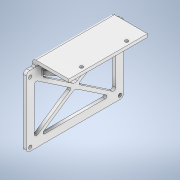
# Autodesk Inventor part: batteryBracket
Saved by Autodesk Inventor 2022 (Build 260153000, 153)
## iProperties
Created: 2022-04-12
Part Number: batteryBracket
Material: PC/ABS Plastic
Document SubType Name: Modeling
Designer: Dahway
Mass: 22.0736 g
Surface Area: 159.209 cm^2
Volume: 22.0736 cm^3
Density: 0.357273 g/cm^3
Appearance: Smooth - White
Author: Dahway
Autodesk Inventor part; units mm, degrees
ref_plane "YZ Plane" through (0, 0, 0) normal (1, 0, 0) x (0, 1, 0)
ref_plane "XZ Plane" through (0, 0, 0) normal (0, 1, 0) x (-1, 0, 0)
ref_plane "XY Plane" through (0, 0, 0) normal (0, 0, 1) x (1, 0, 0)
sketch "Sketch1" plane through (0, 0, 0) normal (0, 1, 0) x (-1, 0, 0)
  line L0 (0, 0) -> (34.8, 0)
  line L1 (34.8, 0) -> (34.8, 75.4)
  line L2 (34.8, 75.4) -> (0, 75.4)
  line L3 (0, 75.4) -> (0, 0)
  dimension "d0" = 34.8
  dimension "d1" = 75.4
  constraints: 8 end point, 2 parallel, 1 horizontal, 1 perpendicular
  measures "d0" distance of L2.end L1.end
  measures "d1" distance of L1.end L0.end
extrude "Extrusion1" add sketch "Sketch1" along normal blind 40.7
sketch "Sketch2" plane through (0, 0, 0) normal (0, -1, 0) x (1, 0, 0)
  line L0 (0, 75.4) -> (0, 0) projected
  line L1 (-34.8, 75.4) -> (0, 75.4) projected
  line L2 (0, 0) -> (-31.8, 0)
  line L3 (-31.8, 0) -> (-31.8, 75.4)
  line L4 (-31.8, 75.4) -> (0, 75.4)
  line L5 (0, 75.4) -> (0, 0)
  dimension "d4" = 31.8
  constraints: 8 end point, 2 parallel, 1 horizontal, 1 perpendicular, 1 point on line
  measures "d4" distance of L3.end L4.end
extrude "Extrusion2" cut sketch "Sketch2" against normal blind 37.7
ref_plane "Work Plane1" through (0, 40.7, 37.7) normal (0, 0, -1) x (-1, 0, 0)
sketch "Sketch4" plane through (0, 37.7, 0) normal (0, -1, 0) x (1, 0, 0)
  circle A0 centre (-4, 3.7) radius 1.5
  circle A1 centre (-4, 6.5) radius 1.5
  line L0 (-5.5, 3.7) -> (-5.5, 6.5)
  line L1 (-2.5, 3.7) -> (-2.5, 6.5)
  line L2 (0, 0) -> (-31.8, 0) projected
  line L3 (0, 75.4) -> (0, 0) projected
  dimension "d17" = 3
  dimension "d18" = 3
  dimension "d19" = 3.7
  dimension "d20" = 4
  dimension "d21" = 2.8
  constraints: 4 end point, 4 point on circle, 2 centre point, 2 tangent, 1 parallel, 1 vertical
  measures "d17" diameter of A0
  measures "d18" diameter of A1
  measures "d19" distance from line of L2 A0.centre
  measures "d20" distance from line of L3 A0.centre
  measures "d21" distance of A1.centre A0.centre
extrude "Extrusion4" add sketch "Sketch4" along normal blind 3
fillet "Fillet1" radius 1 4 edges at (-4, 34.7, 2.2) (-2.5, 34.7, 5.1) (-4, 34.7, 8) (-5.5, 34.7, 5.1)
mirror "Mirror2" about plane through (0, 40.7, 37.7) normal (0, 0, -1) of "Extrusion4", "Fillet1"
sketch "Sketch22" plane through (0, 40.7, 0) normal (0, 1, 0) x (1, 0, 0)
  line L0 (-34.8, -75.4) -> (0, -75.4) projected
  line L1 (-7.8, -72.1) -> (-7.8, -75.4) projected
  line L2 (0, 0) -> (-34.8, 0) projected
  point P0 (-4, -59.3)
  point P1 (-3.9, -16.1)
  point P2 (-7.8, 0)
  dimension "d126" = 16.1
  dimension "d127" = 3.8
  dimension "d128" = 16.1
  measures "d126" distance from line of L0 point (-4, -59.3)
  measures "d127" distance from line of L1 point (-4, -59.3)
  measures "d128" distance from line of L2 point (-3.9, -16.1)
hole "Hole2" at (-4, 40.7, 59.3) at (-3.9, 40.7, 16.1) direction (0, -1, 0) diameter 3.15 depth 3 tip angle 118
sketch "Sketch24" plane through (-34.8, 0, 0) normal (-1, 0, 0) x (0, 0, 1)
  line L0 (84.25, 34.785) -> (-8.85, 34.785)
  line L1 (-8.85, 34.785) -> (-8.85, -32.5)
  line L2 (-8.85, -32.5) -> (84.25, -32.5)
  line L3 (84.25, -32.5) -> (84.25, 34.785)
  point P0 (0, 0)
  dimension "d170" = 93.1
  dimension "d171" = 67.285
  dimension "d172" = 34.785
  dimension "d173" = 8.85
  constraints: 8 end point, 2 parallel, 1 horizontal, 1 perpendicular
  measures "d170" distance of L2.end L1.end
  measures "d171" distance of L1.end L0.end
  measures "d172" distance from line of point (0, 0) L0
  measures "d173" distance from line of point (0, 0) L1
extrude "Extrusion19" add sketch "Sketch24" against normal up to surface (3 mm away)
fillet "Fillet14" radius 3.15 5 edges at (-33.3, 34.785, -8.85) (-34.8, 40.7, 37.7) (-33.3, 34.785, 84.25) (-33.3, -32.5, 84.25) (-33.3, -32.5, -8.85)
sketch "Sketch26" plane through (-34.8, -29.35, -8.85) normal (-1, 0, 0) x (0, 0, 1)
  line L0 (7.5, 54.45) -> (85.6, 54.45)
  line L1 (85.6, 54.45) -> (85.6, 4.45)
  line L2 (85.6, 4.45) -> (7.5, 4.45)
  line L3 (7.5, 4.45) -> (7.5, 54.45)
  line L4 (7.5, 54.45) -> (85.6, 4.45) construction
  line L5 (85.6, 54.45) -> (7.5, 4.45) construction
  line L6 (0, 60.985) -> (0, 0) projected
  line L7 (3.15, -3.15) -> (89.95, -3.15) projected
  point P0 (8.85, 29.35)
  point P1 (46.55, 29.45)
  dimension "d192" = 78.1
  dimension "d193" = 50
  dimension "d194" = 7.5
  dimension "d195" = 7.6
  constraints: 12 end point, 2 midpoint, 2 parallel, 1 horizontal, 1 perpendicular
  measures "d192" distance of L1.end L2.end
  measures "d193" distance of L0.end L1.end
  measures "d194" distance between parallel lines of L6 L3
  measures "d195" distance between parallel lines of L7 L2
extrude "Extrusion20" cut sketch "Sketch26" against normal up to surface (3 mm away)
fillet "Fillet16" radius 3.15 4 edges at (-33.3, 25.1, -1.35) (-33.3, 25.1, 76.75) (-33.3, -24.9, 76.75) (-33.3, -24.9, -1.35)
fillet "Fillet17" radius 1.415 2 edges at (-33.3, 34.785, 75.4) (-33.3, 34.785, 0)
sketch "Sketch30" plane through (-31.8, -29.35, 84.25) normal (1, 0, 0) x (0, 0, -1)
  line L0 (12.2, 62.05) -> (0.1855, 62.05) projected
  line L1 (0, 60.985) -> (0, 0) projected
  line L2 (92.9145, 62.05) -> (80.9, 62.05) projected
  line L3 (93.1, 0) -> (93.1, 60.985) projected
  point P0 (84.25, 29.35)
  point P1 (3.5, 58.55)
  point P2 (89.6, 58.55)
  point P3 (89.6, 0.35)
  point P4 (3.5, 0.35)
  point P5 (92.6652, 62.05)
  dimension "d222" = 3.5
  dimension "d223" = 3.5
  dimension "d224" = 86.1
  dimension "d225" = 58.2
  dimension "d226" = 58.2
  dimension "d227" = 3.5
  dimension "d228" = 86.1
  dimension "d229" = 3.5
  measures "d222" distance from line of L0 point (3.5, 58.55)
  measures "d223" distance from line of point (3.5, 58.55) L1
  measures "d224" distance of point (89.6, 58.55) point (3.5, 58.55)
  measures "d225" distance of point (89.6, 0.35) point (89.6, 58.55)
  measures "d226" distance of point (3.5, 0.35) point (3.5, 58.55)
  measures "d227" distance from line of L2 point (89.6, 58.55)
  measures "d228" distance of point (89.6, 0.35) point (3.5, 0.35)
  measures "d229" distance from line of L3 point (89.6, 0.35)
hole "Hole4" at (-31.8, 29.2, 80.75) at (-31.8, 29.2, -5.35) at (-31.8, -29, -5.35) at (-31.8, -29, 80.75) direction (-1, 0, 0) diameter 3.3 end through all
sketch "Sketch31" plane through (-34.8, -32.5, -5.7) normal (-1, 0, 0) x (0, 0, 1)
  circle A0 centre (0.35, 3.5) radius 1.65 projected
  line L0 (-0.574, 4.867) -> (85.526, 63.067)
  circle A1 centre (86.45, 61.7) radius 1.65 projected
  circle A2 centre (0.35, 3.5) radius 1.65 projected
  line L1 (87.374, 60.333) -> (1.274, 2.133)
  circle A3 centre (0.35, 61.7) radius 1.65 projected
  line L2 (1.274, 63.067) -> (88.0053, 4.4403)
  circle A4 centre (86.45, 3.5) radius 1.65 projected
  circle A5 centre (0.35, 61.7) radius 1.65 projected
  line L3 (-0.574, 60.333) -> (85.526, 2.133)
  point P0 (5.7, 32.5)
  point P1 (43.4, 30.6084)
  point P2 (87.374, 4.867)
  point P3 (46.3463, 32.6)
  point P4 (43.4, 34.5916)
  point P5 (-0.574, 60.333)
  point P6 (40.4537, 32.6)
  point P7 (1.274, 2.133)
  constraints: 8 end point, 6 tangent, 4 point on circle, 8 other
extrude "Extrusion24" add sketch "Sketch31" against normal up to surface (3 mm away) contours A0 L0 L3 L1 | L3 A3 L2 L0 | L0 L2 L1 L3 | L1 L2 A4 L3 | L0 A1 L1 L2
fillet "Fillet21" radius 4 2 edges at (-33.3, -1.8916, 37.7) (-33.3, 2.0916, 37.7)
fillet "Fillet22" radius 2 4 edges at (-33.3, 23.9949, 75.996) (-33.3, -23.7949, 75.996) (-33.3, -23.7949, -0.596) (-33.3, 23.9949, -0.596)
fillet "Fillet23" radius 1.5 6 edges at (-33.3, -24.9, 3.6618) (-33.3, 25.1, 3.6618) (-33.3, 25.1, 71.7382) (-33.3, -24.9, 71.7382) (-33.3, 0.1, 34.7537) (-33.3, 0.1, 40.6463)
sketch "Sketch32" plane through (0, 37.7, 0) normal (0, -1, 0) x (1, 0, 0)
  line L0 (-7.8, 68.9) -> (-11.8, 68.9)
  line L1 (-11.8, 68.9) -> (-11.8, 6.5)
  line L2 (-11.8, 6.5) -> (-7.8, 6.5)
  line L3 (-7.8, 6.5) -> (-7.8, 68.9)
  line L4 (-7.8, 68.9) -> (-11.8, 6.5) construction
  line L5 (-11.8, 68.9) -> (-7.8, 6.5) construction
  circle A0 centre (-4, 59.3) radius 1.575 projected
  line L6 (-31.8, 75.4) -> (0, 75.4) projected
  point P0 (0, 0)
  point P1 (-9.8, 37.7)
  point P2 (-34.7964, 75.4)
  dimension "d243" = 4
  dimension "d244" = 62.4
  dimension "d245" = 3.8
  dimension "d246" = 6.5
  constraints: 12 end point, 2 midpoint, 2 parallel, 1 horizontal, 1 perpendicular
  measures "d243" distance of L2.end L1.end
  measures "d244" distance of L1.end L0.end
  measures "d245" distance from line of A0.centre L3
  measures "d246" distance between parallel lines of L6 L0
extrude "Extrusion25" add sketch "Sketch32" along normal blind 2 contours L3 L2 L1 L0
fillet "Fillet24" radius 2.915 1 edges at (-31.8, 37.7, 37.7)
sketch "Sketch33" plane through (-11.8, 37.7, 68.9) normal (0, 0, 1) x (1, 0, 0)
  line L0 (4, 0) -> (4, -2) projected
  line L1 (4, -2) -> (-20, -12.6)
  line L2 (0, 0) -> (-20, -8.8333)
  line L3 (0, 0) -> (0, -2) projected
  line L4 (-17.085, 0) -> (11.8, 0) projected
  line L5 (-20, -12.6) -> (-20, -8.8333)
  line L6 (4, -2) -> (0, 0)
  point P0 (11.8, -37.7)
  constraints: 8 end point, 2 point on line, 1 parallel, 1 vertical
extrude "Extrusion26" add sketch "Sketch33" against normal blind 4 contours L1 L5 L2 L6
mirror "Mirror7" about plane through (0, 40.7, 37.7) normal (0, 0, -1) of "Extrusion26"
fillet "Fillet25" radius 3 2 edges at (-7.8, 36.7, 68.9) (-7.8, 36.7, 6.5)
fillet "Fillet27" radius 1 12 edges at (-9.8, 35.7, 64.9) (-9.8, 35.7, 10.5) (-11.8, 36.7, 10.5) (-11.8, 36.7, 64.9) (-11.8, 37.7, 66.9) (-11.8, 37.7, 8.5) (-31.8, 26.9833, 6.5) (-31.8, 28.8667, 8.5) (-31.8, 26.9833, 10.5) (-31.8, 26.9833, 64.9) (-31.8, 28.8667, 66.9) (-31.8, 26.9833, 68.9)
body "Solid1"
